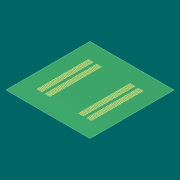
# Autodesk Inventor part: backerConnectorMount
Saved by Autodesk Inventor 2016 (Build 200138000, 138)
## iProperties
Created: 2016-06-07
Part Number: backerConnectorMount
Material: ABS Plastic
Document SubType Name: Modeling
Designer: sawaiz
Density: 1.06 g/cm^3
Appearance: Smooth - Dark Sea Green
Author: sawaiz
Autodesk Inventor part; units mm, degrees
ref_plane "YZ Plane" through (0, 0, 0) normal (1, 0, 0) x (0, 1, 0)
ref_plane "XZ Plane" through (0, 0, 0) normal (0, 1, 0) x (-1, 0, 0)
ref_plane "XY Plane" through (0, 0, 0) normal (0, 0, 1) x (1, 0, 0)
sketch "Sketch1" plane through (0, 0, 0) normal (0, 1, 0) x (-1, 0, 0)
  line L0 (12.9, 12.9) -> (-12.9, 12.9)
  line L1 (-12.9, 12.9) -> (-12.9, -12.9)
  line L2 (-12.9, -12.9) -> (12.9, -12.9)
  line L3 (12.9, -12.9) -> (12.9, 12.9)
  line L4 (12.9, 12.9) -> (-12.9, -12.9) construction
  line L5 (-12.9, 12.9) -> (12.9, -12.9) construction
  point P0 (0, 0)
  dimension "d0" = 25.8
  dimension "d1" = 25.8
  constraints: 12 end point, 2 midpoint, 2 parallel, 1 horizontal, 1 perpendicular
  measures "d0" distance of L2.end L1.end
  measures "d1" distance of L1.end L0.end
extrude "Extrusion1" add sketch "Sketch1" along normal blind 0.01
sketch "Sketch3" plane through (0, 0, 0) normal (0, -1, 0) x (1, 0, 0)
  line L0 (6.9, -0.075) -> (8.4, -0.075)
  line L1 (8.4, -0.075) -> (8.4, -0.325)
  line L2 (8.4, -0.325) -> (6.9, -0.325)
  line L3 (6.9, -0.325) -> (6.9, -0.075)
  line L4 (6.9, -0.075) -> (8.4, -0.325) construction
  line L5 (8.4, -0.075) -> (6.9, -0.325) construction
  line L6 (5.9, -0.075) -> (4.4, -0.075)
  line L7 (4.4, -0.075) -> (4.4, -0.325)
  line L8 (4.4, -0.325) -> (5.9, -0.325)
  line L9 (5.9, -0.325) -> (5.9, -0.075)
  line L10 (5.9, -0.075) -> (4.4, -0.325) construction
  line L11 (4.4, -0.075) -> (5.9, -0.325) construction
  point P0 (0, 0)
  point P1 (7.65, -0.2)
  point P2 (5.15, -0.2)
  dimension "d24" = 0.25
  dimension "d25" = 1.5
  dimension "d26" = 6.9
  dimension "d27" = 0.325
  dimension "d33" = 1.5
  dimension "d34" = 4
  constraints: 24 end point, 4 midpoint, 4 parallel, 2 collinear, 2 horizontal, 2 perpendicular
  measures "d24" distance of L0.end L1.end
  measures "d25" distance of L1.end L2.end
  measures "d26" distance from line of point (0, 0) L3
  measures "d27" distance from line of point (0, 0) L2
  measures "d33" distance of L7.end L8.end
  measures "d34" distance between parallel lines of L1 L7
extrude "Extrusion3" add sketch "Sketch3" along normal blind 0.01 separate body
pattern_linear "Rectangular Pattern3" count 20 spacing 0.4 along (0, 0, -1) of "Extrusion3" bodies 2
pattern_linear "Rectangular Pattern4" count 2 spacing 8 along (0, 0, 1) of "Extrusion3", "Rectangular Pattern3" bodies 2
mirror "Mirror1" about plane through (0, 0, 0) normal (1, 0, 0) of "Extrusion3", "Rectangular Pattern3", "Rectangular Pattern4" bodies 2
body "Solid1"
body "Solid3"
